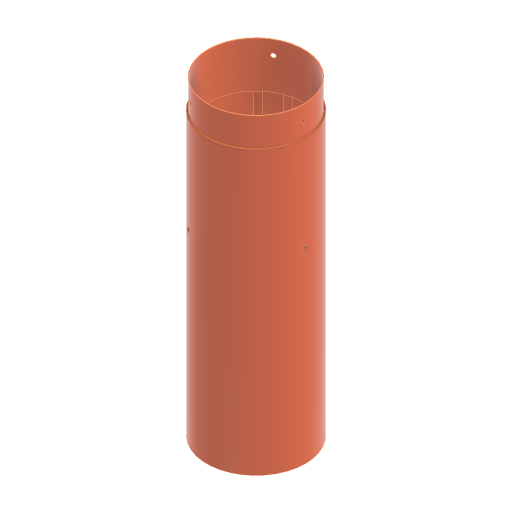
# Autodesk Inventor part: Lower skin
Saved by Autodesk Inventor 2024 (Build 280153000, 153)
## iProperties
Created: 2023-12-30
Part Number: Lower skin
Material: Plastic, Opaque White
Document SubType Name: Modeling
Designer: Jamie
Density: 0.952 g/cm^3
Appearance: Smooth - Light Orange
Author: Jamie
Autodesk Inventor part; units mm, degrees
ref_plane "XZ Plane" through (0, 0, 0) normal (0, 1, 0) x (-1, 0, 0)
ref_plane "XY Plane" through (0, 0, 0) normal (0, 0, 1) x (1, 0, 0)
sketch "Sketch1" plane through (0, 0, 0) normal (0, 1, 0) x (-1, 0, 0)
  circle A0 centre (0, 0) radius 35
  circle A1 centre (0, 0) radius 34.5
  dimension "d0" = 70
  dimension "d1" = 69
  constraints: 2 centre point, 2 coincident
  measures "d0" diameter of A0
  measures "d1" diameter of A1
extrude "Extrusion1" add sketch "Sketch1" along normal blind 200
ref_plane "Work Plane2" through (35, 0, 0) normal (1, 0, 0) x (0, 1, 0)
sketch "Sketch4" plane through (35, 0, 0) normal (1, 0, 0) x (0, 1, 0)
  line L0 (200, -35) -> (200, 35) projected
  point P0 (0, 0)
  point P1 (132.5, 0)
  dimension "d48" = 132.5
  measures "d48" distance of point (0, 0) point (132.5, 0)
hole "Hole2" at (35, 132.5, 0) direction (-1, 0, 0) diameter 3 depth 8 tip angle 118
sketch "Sketch5" plane through (0, 200, 0) normal (0, 1, 0) x (1, 0, 0)
  circle A0 centre (0, 0) radius 34
  circle A1 centre (0, 0) radius 33.5
  dimension "d44" = 68
  dimension "d45" = 67
  constraints: 2 centre point, 2 coincident
  measures "d44" diameter of A0
  measures "d45" diameter of A1
extrude "Extrusion3" add sketch "Sketch5" along normal blind 20
sketch "Sketch6" plane through (0, 200, 0) normal (0, -1, 0) x (1, 0, 0)
  circle A0 centre (0, 0) radius 33.5
  circle A1 centre (0, 0) radius 34.5 projected
  circle A2 centre (0, 0) radius 35
  constraints: 2 centre point, 2 coincident
extrude "Extrusion4" add sketch "Sketch6" along normal blind 12.5 contours A1
ref_plane "Work Plane4" through (34, 0, 0) normal (1, 0, 0) x (0, 1, 0)
sketch "Sketch8" plane through (34, 0, 0) normal (1, 0, 0) x (0, 1, 0)
  line L0 (220, -34) -> (220, 34) projected
  point P0 (0, 0)
  point P1 (210, 0)
  dimension "d61" = 10
  measures "d61" distance from line of L0 point (210, 0)
hole "Hole4" at (34, 210, 0) direction (-1, 0, 0) diameter 3 depth 8 tip angle 118
pattern_circular "Circular Pattern2" count 3 over 360 about axis through (0, 0, 0) along (0, 1, 0) of "Hole2", "Hole4"
sketch "Sketch9" plane through (0, 0, 0) normal (0, -1, 0) x (1, 0, 0)
  line L0 (34.0588, 0) -> (34.0588, -5.5) construction
  circle A0 centre (0, 0) radius 34.5 projected
  line L1 (34.0588, -5.5) -> (33.0454, -5.5)
  circle A1 centre (0, 0) radius 33.5 projected
  line L2 (33.0454, -5.5) -> (33.0454, -9.9121)
  arc A2 (33.0454, -9.9121) -> (34.0588, -5.5) centre (0, 0) ccw
  dimension "d72" = 5.5
  dimension "d73" = 0
  constraints: 6 end point, 4 point on circle, 2 vertical, 1 centre point, 1 coincident, 1 horizontal, 2 other
  measures "d72" distance of L0.start L0.end
  measures "d73" vertical distance of point (0, 0) L0.start
extrude "Extrusion5" add sketch "Sketch9" against normal blind 200 contours L2 L1 A0 picked at (33.1794, -7.9563)
mirror "Mirror1" about plane through (0, 0, 0) normal (0, 0, 1) of "Extrusion5"
pattern_circular "Circular Pattern3" count 3 over 360 about axis through (0, 0, 0) along (0, 1, 0) of "Extrusion5", "Mirror1"
body "Solid1"
